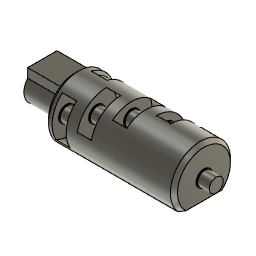
mmu2-idler-heated-inserts (Autodesk Fusion 360 design; units mm, degrees)
Autodesk Fusion 360 part; units mm, degrees
sketch "bottom idler" plane through (0, 0, 0) normal (1, 0, 0) x (0, 1, 0)
  line L0 (-2.2115, -1.832) -> (-2.137, -1.9113)
  line L1 (2.6836, -0.9917) -> (2.7236, -0.8905)
  line L2 (1.2798, -2.5631) -> (1.3783, -2.5168)
  line L3 (-2.2755, 1.7345) -> (-2.4231, 1.5314)
  line L4 (-2.4231, 1.5314) -> (-2.5441, 1.3113)
  line L5 (1.2484, 2.5685) -> (1.0526, 2.6607)
  line L6 (-2.8637, -0.1847) -> (-2.8501, -0.2927)
  line L7 (-0.8192, -2.7477) -> (-0.7156, -2.7813)
  line L8 (-2.8186, -0.5418) -> (-2.7562, -0.7851)
  line L9 (2.7507, -0.7851) -> (2.8132, -0.5418)
  line L10 (-1.3838, 2.5074) -> (-1.4757, 2.4491)
  line L11 (-1.3838, -2.5168) -> (-1.2853, -2.5631)
  line L12 (0.6033, 2.7923) -> (0.3565, 2.8394)
  line L13 (-1.8812, -2.1638) -> (-1.6877, -2.3239)
  line L14 (-0.7156, -2.7813) -> (-0.6087, -2.8017)
  line L15 (2.8546, -0.2136) -> (1.2484, 2.5685)
  line L16 (1.6822, -2.3239) -> (1.8758, -2.1638)
  line L17 (-2.689, 0.9824) -> (-2.7291, 0.8812)
  line L18 (-2.689, -0.9917) -> (-2.5966, -1.2253)
  line L19 (-0.6087, -2.8017) -> (-0.362, -2.8487)
  line L20 (2.8446, -0.2927) -> (2.8546, -0.2136)
  line L21 (2.8854, -0.2669) -> (1.2154, 2.627)
  line L22 (0.7102, 2.7719) -> (0.6033, 2.7923)
  line L23 (-0.8192, 2.7383) -> (-1.058, 2.6607)
  line L24 (2.4177, -1.5407) -> (2.5387, -1.3206)
  line L25 (-1.2853, 2.5537) -> (-1.3838, 2.5074)
  line L26 (1.4702, -2.4584) -> (1.6822, -2.3239)
  line L27 (-2.5441, -1.3206) -> (-2.4231, -1.5407)
  line L28 (-0.1114, 2.8551) -> (-0.362, 2.8394)
  line L29 (2.1316, -1.9113) -> (2.2061, -1.832)
  line L30 (-2.8637, 0.1753) -> (-2.8637, -0.1847)
  line L31 (1.0526, 2.6607) -> (0.8137, 2.7383)
  line L32 (-2.8186, 0.5325) -> (-2.8501, 0.2833)
  line L33 (-2.5966, -1.2253) -> (-2.5441, -1.3206)
  line L34 (-2.7291, -0.8905) -> (-2.689, -0.9917)
  line L35 (-1.4757, 2.4491) -> (-1.6877, 2.3145)
  line L36 (2.7236, -0.8905) -> (2.7507, -0.7851)
  line L37 (-0.6087, 2.7923) -> (-0.7156, 2.7719)
  line L38 (1.3783, -2.5168) -> (1.4702, -2.4584)
  line L39 (-2.7291, 0.8812) -> (-2.7562, 0.7757)
  line L40 (-0.7156, 2.7719) -> (-0.8192, 2.7383)
  line L41 (-1.6877, 2.3145) -> (-1.8812, 2.1544)
  line L42 (-2.8501, 0.2833) -> (-2.8637, 0.1753)
  line L43 (0.3565, 2.8394) -> (0.1059, 2.8551)
  line L44 (2.2061, -1.832) -> (2.27, -1.7439)
  line L45 (-1.8812, 2.1544) -> (-1.9651, 2.085)
  line L46 (2.5387, -1.3206) -> (2.5911, -1.2253)
  line L47 (-2.5441, 1.3113) -> (-2.5966, 1.2159)
  line L48 (2.8132, -0.5418) -> (2.8446, -0.2927)
  line L49 (0.8137, 2.7383) -> (0.7102, 2.7719)
  line L50 (2.5911, -1.2253) -> (2.6836, -0.9917)
  line L51 (-2.7562, -0.7851) -> (-2.7291, -0.8905)
  line L52 (-1.9651, 2.085) -> (-2.137, 1.9019)
  line L53 (1.0526, -2.67) -> (1.2798, -2.5631)
  line L54 (0.7102, -2.7813) -> (0.8137, -2.7477)
  line L55 (2.27, -1.7439) -> (2.4177, -1.5407)
  line L56 (0.1059, 2.8551) -> (-0.0027, 2.862)
  line L57 (-2.2115, 1.8226) -> (-2.2755, 1.7345)
  line L58 (1.9596, -2.0944) -> (2.1316, -1.9113)
  line L59 (-2.5966, 1.2159) -> (-2.689, 0.9824)
  line L60 (-1.058, 2.6607) -> (-1.2853, 2.5537)
  line L61 (0.8137, -2.7477) -> (1.0526, -2.67)
  line L62 (-2.4231, -1.5407) -> (-2.2755, -1.7439)
  line L63 (-0.362, 2.8394) -> (-0.6087, 2.7923)
  line L64 (1.8758, -2.1638) -> (1.9596, -2.0944)
  line L65 (-2.8501, -0.2927) -> (-2.8186, -0.5418)
  line L66 (-2.7562, 0.7757) -> (-2.8186, 0.5325)
  line L67 (-2.137, 1.9019) -> (-2.2115, 1.8226)
  line L68 (-0.0027, 2.862) -> (-0.1114, 2.8551)
  line L69 (14.217, 3.3662) -> (9.8122, 10.9953)
  circle A0 centre (-0.0027, -0.0047) radius 2.9
  line L70 (0.6033, -2.8017) -> (0.7102, -2.7813)
  line L71 (-1.9651, -2.0944) -> (-1.8812, -2.1638)
  line L72 (9.8122, 10.9953) -> (14.217, 3.3662)
  arc A1 (8.7943, -1.8539) -> (-6.8329, 5.8386) centre (0, 0) cw
  line L73 (12.4076, 0.2322) -> (8.7943, -1.8539)
  line L74 (12.4076, 0.2322) -> (14.217, 3.3662)
  line L75 (0.1059, -2.8645) -> (0.3565, -2.8487)
  line L76 (8.7943, -1.8539) -> (12.4076, 0.2322)
  line L77 (-6.8329, 5.8386) -> (-6.8329, 10.9953)
  line L78 (-1.6877, -2.3239) -> (-1.4757, -2.4584)
  line L79 (0.3565, -2.8487) -> (0.6033, -2.8017)
  line L80 (-2.2755, -1.7439) -> (-2.2115, -1.832)
  line L81 (14.217, 3.3662) -> (12.4076, 0.2322)
  line L82 (-0.0027, -2.8714) -> (0.1059, -2.8645)
  line L83 (-6.8329, 10.9953) -> (-6.8329, 5.8386)
  line L84 (-2.137, -1.9113) -> (-1.9651, -2.0944)
  line L85 (-0.1114, -2.8645) -> (-0.0027, -2.8714)
  line L86 (-1.2853, -2.5631) -> (-1.058, -2.67)
  line L87 (9.8122, 10.9953) -> (-6.8329, 10.9953)
  line L88 (-1.4757, -2.4584) -> (-1.3838, -2.5168)
  line L89 (-0.362, -2.8487) -> (-0.1114, -2.8645)
  line L90 (-1.058, -2.67) -> (-0.8192, -2.7477)
  circle A2 centre (0, 0) radius 8.9876
  line L91 (-6.8329, 10.9953) -> (9.8122, 10.9953)
sketch "Sketch15" plane through (0, 0, 0) normal (0, 1, 0) x (1, 0, 0)
extrude "Extrude1" add sketch "bottom idler" along normal blind 20 contours L15 L21 A0 | L69 L72 L73 L74 L76 L77 L81 L83 L87 A2 L91 | A1 A2 makes body 1
sketch "Sketch17" plane through (0, 12.1203, 6.9977) normal (0, 0.866023, 0.500004) x (-1, 0, 0)
  line L0 (0, -4.1934) -> (0, 4.616)
  line L1 (0, 4.616) -> (-20, 4.616)
  line L2 (-20, 4.616) -> (-20, -4.1934)
  line L3 (-20, -4.1934) -> (0, -4.1934)
  line L4 (-19.7165, 4.3663) -> (-10, -4.1934) construction
  line L5 (-10, -4.1934) -> (0, 4.616) construction
  circle A0 centre (-14.8583, 0.0865) radius 2.85
  circle A1 centre (-5.2702, -0.0267) radius 2.85
  circle A2 centre (-14.8583, 0.0865) radius 1.6
  circle A3 centre (-5.2702, -0.0267) radius 1.6
  circle A4 centre (-14.8583, 0.0865) radius 2.3
  circle A5 centre (-5.2702, -0.0267) radius 2.3
  dimension "d58" = 5.7
  dimension "d59" = 5.7
  dimension "d60" = 3.2
  dimension "d61" = 3.2
  dimension "d62" = 4.6
  dimension "d63" = 4.6
  constraint midpoint L3 L4.end
  constraint midpoint L4 A0.centre
  constraint concentric A0 A2
  constraint concentric A1 A3
  constraint concentric A2 A4
  constraint concentric A3 A5
  measures "d58" diameter of A0
  measures "d59" diameter of A1
  measures "d60" diameter of A2
  measures "d61" diameter of A3
  measures "d62" diameter of A4
  measures "d63" diameter of A5
extrude "Extrude17" cut sketch "Sketch17" against normal blind 4 contours A0 | A1 | A2 | A3 | A4 | A5 bodies 1
extrude "Extrude18" cut sketch "Sketch17" against normal blind 14 contours A2 | A3 bodies 1
extrude "Extrude19" cut sketch "Sketch17" against normal blind 10 contours A4 | A5 bodies 1
sketch "Sketch14" plane through (0, 0, 0) normal (-1, 0, 0) x (0, -1, 0)
  circle A0 centre (-0.0027, -0.0047) radius 8.9876
  line L0 (-8.797, 1.8492) -> (-12.4103, -0.2369)
  line L1 (-12.4103, -0.2369) -> (-14.2197, -3.3708)
  line L2 (-14.2197, -3.3708) -> (-9.815, -11)
  line L3 (-9.815, -11) -> (6.8301, -11)
  line L4 (6.8301, -11) -> (6.8301, -5.8432)
  circle A1 centre (0, 0) radius 2.9
  line L5 (-2.8881, 0.2622) -> (-1.2182, -2.6317)
  arc A2 (-8.7943, -1.8539) -> (6.8329, 5.8386) centre (0, 0) ccw
  line L6 (6.8329, 5.8386) -> (6.8329, 10.9953)
  line L7 (6.8329, 10.9953) -> (-9.8122, 10.9953)
  line L8 (-9.8122, 10.9953) -> (-14.217, 3.3662)
  line L9 (-14.217, 3.3662) -> (-12.4076, 0.2322)
  line L10 (-12.4076, 0.2322) -> (-8.7943, -1.8539)
  line L11 (-2.8854, -0.2669) -> (-1.2154, 2.627)
  arc A3 (-2.8854, -0.2669) -> (-1.2154, 2.627) centre (0.0027, -0.0047) ccw
  constraint coincident A1.centre A2.centre
sketch "Sketch6" plane through (20, 0, 0) normal (1, 0, 0) x (0, 1, 0)
  circle A0 centre (0, 0) radius 2.9
  line L0 (2.8881, 0.2622) -> (1.2182, -2.6317)
  arc A1 (-6.8329, 5.8386) -> (8.7943, -1.8539) centre (0, 0) ccw
  line L1 (8.7943, -1.8539) -> (12.4076, 0.2322)
  line L2 (12.4076, 0.2322) -> (14.217, 3.3662)
  line L3 (14.217, 3.3662) -> (9.8122, 10.9953)
  line L4 (9.8122, 10.9953) -> (-6.8329, 10.9953)
  line L5 (-6.8329, 10.9953) -> (-6.8329, 5.8386)
  line L6 (1.2154, 2.627) -> (2.8854, -0.2669)
  arc A2 (1.2154, 2.627) -> (2.8854, -0.2669) centre (-0.0027, -0.0047) ccw
  dimension "d21" = 5.8
  constraint coincident A0.centre A1.centre
  constraint coincident A0 L0.start
  constraint coincident A0 L0.end
  measures "d21" diameter of A0
extrude "Extrude8" cut sketch "Sketch6" against normal blind 20 contours A0 L0 L6 | A0 L0 L6 A2 picked at (1.8494, 1.6828) picked at (1.448, 1.8318) bodies 1
sketch "Sketch7" plane through (20, 0, 0) normal (1, 0, 0) x (0, 1, 0)
  circle A0 centre (0, 0) radius 17
  arc A1 (-6.8329, 5.8386) -> (8.7943, -1.8539) centre (0, 0) ccw
  line L0 (8.7943, -1.8539) -> (12.4076, 0.2322)
  line L1 (12.4076, 0.2322) -> (14.217, 3.3662)
  line L2 (14.217, 3.3662) -> (9.8122, 10.9953)
  line L3 (9.8122, 10.9953) -> (-6.8329, 10.9953)
  line L4 (-6.8329, 10.9953) -> (-6.8329, 5.8386)
  line L5 (2.8881, 0.2622) -> (2.7341, -0.0047)
  line L6 (2.7341, -0.0047) -> (2.8854, -0.2669)
  arc A2 (-2.5057, 1.4599) -> (2.8854, -0.2669) centre (-0.0027, -0.0047) ccw
  arc A3 (2.8881, 0.2622) -> (-2.5057, 1.4599) centre (0, 0) ccw
  constraint coincident A0.centre A1.centre
extrude "Extrude9" add sketch "Sketch7" along normal blind 73 contours A0 | A1 L0 L1 L2 L3 L4 | L5 L6 A2 A3 bodies 1
sketch "Sketch8" plane through (20, 0, 0) normal (-1, 0, 0) x (0, -1, 0)
  circle A0 centre (0, 0) radius 17
  circle A1 centre (0, 0) radius 15.5
  line L0 (-3.972, -11) -> (-3.972, 16.5295)
  line L1 (-12.9615, -11) -> (12.9615, -11)
  line L2 (6.8329, 10.9953) -> (6.8329, 5.8386)
  arc A2 (-8.7943, -1.8539) -> (6.8329, 5.8386) centre (0, 0) ccw
  line L3 (-8.7943, -1.8539) -> (-12.4076, 0.2322)
  line L4 (-12.4076, 0.2322) -> (-14.217, 3.3662)
  line L5 (-14.217, 3.3662) -> (-9.8122, 10.9953)
  line L6 (-9.8122, 10.9953) -> (6.8329, 10.9953)
  constraint coincident A0 L0.end
  constraint vertical L0
  constraint coincident A0 L1.start
  constraint coincident A0 L1.end
  constraint perpendicular L0 L1
extrude "Extrude10" cut sketch "Sketch8" against normal blind 110 contours A0 A1 L1 | A1 L1 bodies 1
extrude "Extrude11" cut sketch "Sketch8" along normal blind 6 from surface at -12.7 contours A0 A1 L0 L1 picked at (-13.2436, -9.7903) bodies 1
sketch "Sketch10" plane through (0, 0, 0) normal (-1, 0, 0) x (0, -1, 0)
  line L0 (0, 0) -> (16.7417, 2.952)
  line L1 (0, 0) -> (17, 0) construction
  line L2 (0, 0) -> (8.8633, 1.5628)
  circle A0 centre (8.8633, 1.5628) radius 11.5
  circle A1 centre (8.8633, 1.5628) radius 3.95
  arc A2 (-8.7943, -1.8539) -> (6.8329, 5.8386) centre (0, 0) ccw
  line L3 (6.8329, 5.8386) -> (6.8329, 10.9953)
  line L4 (-9.8122, 10.9953) -> (-14.217, 3.3662)
  line L5 (-14.217, 3.3662) -> (-12.4076, 0.2322)
  line L6 (-12.4076, 0.2322) -> (-8.7943, -1.8539)
  line L7 (6.8329, 10.9953) -> (-9.8122, 10.9953)
  line L8 (-2.7341, -0.0047) -> (-2.8881, 0.2622)
  arc A3 (2.5057, 1.4599) -> (-2.8881, 0.2622) centre (0, 0) ccw
  arc A4 (-2.8854, -0.2669) -> (2.5057, 1.4599) centre (0.0027, -0.0047) ccw
  line L9 (-2.8854, -0.2669) -> (-2.7341, -0.0047)
  dimension "d35" = 10
  dimension "d36" = 17
  dimension "d37" = 9
  dimension "d39" = 23
  dimension "d40" = 7.9
  constraint horizontal L1
  constraint coincident L0.start L1.start
  constraint coincident L0 L2.end
  constraint coincident L2.end A0.centre
  constraint concentric A0 A1
  measures "d35" angle of L0 L1
  measures "d36" distance of L0.start L0.end
  measures "d37" distance of L0.start L2.end
  measures "d39" diameter of A0
  measures "d40" diameter of A1
extrude "Extrude12" add sketch "Sketch10" against normal blind 8 separate body contours L0 L2 A0 A1 A2 L3 L7 A3 A4 | L0 L2 A0 A1 A2 A4 | A0 A3 A4 | A0 A1 A2 L3 L7 makes body 2
sketch "Sketch11" plane through (0, 0, 0) normal (-1, 0, 0) x (0, -1, 0)
  circle A0 centre (8.8633, 1.5628) radius 3.95
  circle A1 centre (8.8633, 1.5628) radius 11.5
  circle A2 centre (8.8633, 1.5628) radius 4.5
  dimension "d45" = 9
  constraint concentric A0 A2
  measures "d45" diameter of A2
extrude "Extrude13" cut sketch "Sketch11" against normal blind 0.4 contours A2 bodies 2
sketch "Sketch12" plane through (8, 0, 0) normal (1, 0, 0) x (0, 1, 0)
  circle A0 centre (-8.8633, 1.5628) radius 3.95
  circle A1 centre (-8.8633, 1.5628) radius 11.5
  circle A2 centre (-8.8633, 1.5628) radius 4.5
  dimension "d48" = 9
  constraint concentric A0 A2
  measures "d48" diameter of A2
extrude "Extrude14" cut sketch "Sketch12" against normal blind 0.4 contours A2 bodies 2
move_body "Move1" bodies 2 to x (1, 0, 0) y (0, 1, 0) z (0, 0, 1) at (19, 0, 0)
pattern_circular "C-Pattern1" count 5 over 160 about axis through (1.75, 0, 0) along (-1, 0, 0) of bodies 2 makes body 3 at (24.3333, -15.2868, 13.3726) makes body 4 at (24.3333, -3.1147, 20.0702) makes body 5 at (24.3333, 10.5149, 17.3767) makes body 6 at (24.3333, 19.2244, 6.5525)
move_face "MoveFace1" to x (1, 0, 0) y (0, 1, 0) z (0, 0, 1) at (5, 0, 0) 1 faces at (24.3333, -20.3061, 0.4178) on bodies 2
move_body "Move2" bodies 2 to x (1, 0, 0) y (0, 1, 0) z (0, 0, 1) at (5, 0, 0)
move_body "Move3" bodies 3 to x (1, 0, 0) y (0, 1, 0) z (0, 0, 1) at (19, 0, 0)
move_face "MoveFace2" to x (1, 0, 0) y (0, 1, 0) z (0, 0, 1) at (33, 0, 0) 1 faces at (24.3333, -3.1147, 20.0702) on bodies 4
move_body "Move4" bodies 4 to x (1, 0, 0) y (0, 1, 0) z (0, 0, 1) at (33, 0, 0)
move_body "Move5" bodies 5 to x (1, 0, 0) y (0, 1, 0) z (0, 0, 1) at (47, 0, 0)
move_body "Move6" bodies 6 to x (1, 0, 0) y (0, 1, 0) z (0, 0, 1) at (61, 0, 0)
combine "Combine1" operation cut target body 1 tool bodies 5 4 3 2 6
sketch "Sketch13" plane through (93, 0, 0) normal (1, 0, 0) x (0, 1, 0)
  line L0 (-12.9615, -11) -> (12.9615, -11)
  arc A0 (12.9615, -11) -> (-12.9615, -11) centre (0, 0) ccw
  circle A1 centre (0, 0) radius 3.95
  circle A2 centre (0, 0) radius 4.5
  dimension "d51" = 7.9
  dimension "d54" = 9
  constraint coincident A0.centre A1.centre
  measures "d51" diameter of A1
  measures "d54" diameter of A2
extrude "Extrude16" add sketch "Sketch13" along normal blind 0.4 contours A2 bodies 1
extrude "Extrude15" add sketch "Sketch13" along normal blind 7 contours A1 bodies 1
chamfer "Chamfer1" distance 2 angle 45 2 edges at (93, 0, 17) (20, 0, 17) on bodies 1
fillet "Fillet1" radius 0.3 2 edges at (7.4145, 8.2536, 5.6949) (17.0026, 8.1971, 5.7929) on bodies 1
chamfer "Chamfer2" distance 1.5 angle 45 2 edges at (26.7, 16.1603, 5.277) (32.7, 16.1603, 5.277) on bodies 1
equation "d26 = -endstopgroove"
equation "endstopgroove = 1.5 mm"
equation "endstoppositionfrombottom = 12.70 mm"
equation "d31 = endstopheight"
equation "endstopheight = 6 mm"
equation "d34 = -endstoppositionfrombottom"
equation "d37 = idlerbearingdistancefromcenter"
equation "idlerbearingdistancefromcenter = 9 mm"
equation "d68 = -4 mm - 6 mm"
